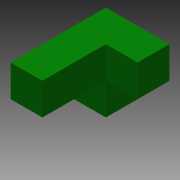
# Autodesk Inventor part: Green Puzzle Cube
Saved by Autodesk Inventor 2015 (Build 190159000, 159)
## iProperties
Created: 2017-11-16
Part Number: Green Puzzle Cube
Material: Generic
Document SubType Name: Modeling
Designer: Administrator
Density: 1 g/cm^3
Appearance: Default
Author: Administrator
Autodesk Inventor part; units mm, degrees
ref_plane "YZ Plane" through (0, 0, 0) normal (1, 0, 0) x (0, 1, 0)
ref_plane "XZ Plane" through (0, 0, 0) normal (0, 1, 0) x (-1, 0, 0)
ref_plane "XY Plane" through (0, 0, 0) normal (0, 0, 1) x (1, 0, 0)
sketch "Sketch1" plane through (0, 0, 0) normal (0, 1, 0) x (-1, 0, 0)
  line L0 (0, 57.15) -> (-19.05, 57.15)
  line L1 (-19.05, 57.15) -> (-19.05, 19.05)
  line L2 (-19.05, 19.05) -> (-38.1, 19.05)
  line L3 (-38.1, 19.05) -> (-38.1, 0)
  line L4 (-38.1, 0) -> (0, 0)
  line L5 (0, 0) -> (0, 57.15)
  dimension "d0" = 57.15
  dimension "d1" = 38.1
  dimension "d2" = 19.05
  dimension "d3" = 19.05
  dimension "d4" = 38.1
  dimension "d5" = 19.05
  constraints: 12 end point, 3 perpendicular, 1 horizontal
  measures "d0" distance of L4.end L0.start
  measures "d1" distance of L3.end L4.end
  measures "d2" distance of L0.start L0.end
  measures "d3" distance of L2.end L3.end
  measures "d4" distance of L0.end L1.end
  measures "d5" distance of L1.end L2.end
extrude "Extrusion1" add sketch "Sketch1" along normal blind 19.05
sketch "Sketch2" plane through (0, 0, 0) normal (0, -1, 0) x (1, 0, 0)
  line L0 (0, 0) -> (0, 57.15) projected
  line L1 (0, 19.05) -> (19.05, 19.05)
  line L2 (19.05, 19.05) -> (19.05, 0)
  line L3 (19.05, 0) -> (0, 0)
  line L4 (0, 0) -> (0, 19.05)
  constraints: 8 end point, 2 perpendicular, 1 collinear, 1 horizontal, 1 point on line
extrude "Extrusion2" add sketch "Sketch2" along normal blind 19.05
body "Solid1"
